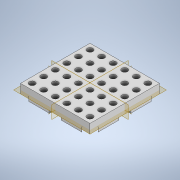
# Autodesk Inventor part: Tile
Saved by Autodesk Inventor 2022.4 (Build 264492010, 492A)
## iProperties
Created: 2025-02-20
Part Number: Tile
Material: Generic
Document SubType Name: Modeling
Designer: jan-m
Density: 1 g/cm^3
Appearance: Default
Author: jan-m
Autodesk Inventor part; units mm, degrees
sketch "Sketch1" plane through (0, 0, 0) normal (0, 1, 0) x (-1, 0, 0)
  line L0 (30, -30) -> (-30, -30)
  line L1 (-30, -30) -> (-30, 30)
  line L2 (-30, 30) -> (30, 30)
  line L3 (30, 30) -> (30, -30)
  line L4 (0, -42) -> (0, 42) projected
  line L5 (-42, 0) -> (42, 0) projected
  point P0 (0, 0)
  point P1 (0, -30)
  point P2 (30, 0)
  dimension "d0" = 60
  dimension "d1" = 60
  constraints: 8 end point, 2 midpoint, 2 parallel, 2 point on line, 1 horizontal, 1 perpendicular
  measures "d0" distance of L0.start L0.end
  measures "d1" distance of L2.end L0.start
extrude "Extrusion1" add sketch "Sketch1" along normal mid plane 10
sketch "Sketch2" plane through (0, -5, 0) normal (0, -1, 0) x (1, 0, 0)
  line L0 (-30, -30) -> (-30, 30) projected
  line L1 (-30, 5) -> (-22, 5)
  line L2 (-22, 5) -> (-22, -5)
  line L3 (-22, -5) -> (-30, -5)
  line L4 (-30, -5) -> (-30, 5)
  arc A0 (-22, -5) -> (-22, 5) centre (-22, 0) ccw
  line L5 (-53.2, 0) -> (53.2, 0) projected
  line L6 (-25, 5) -> (-25, -5)
  line L7 (0, -53.2) -> (0, 53.2) projected
  line L8 (-5, -30) -> (-5, -22)
  arc A1 (5, -22) -> (-5, -22) centre (0, -22) ccw
  line L9 (5, -22) -> (5, -30)
  line L10 (5, -30) -> (-5, -30)
  line L11 (-5, -25) -> (5, -25)
  line L12 (-5, -22) -> (5, -22)
  line L13 (30, -5) -> (22, -5)
  arc A2 (22, 5) -> (22, -5) centre (22, 0) ccw
  line L14 (22, 5) -> (30, 5)
  line L15 (30, 5) -> (30, -5)
  line L16 (25, -5) -> (25, 5)
  line L17 (22, -5) -> (22, 5)
  line L18 (5, 30) -> (5, 22)
  arc A3 (-5, 22) -> (5, 22) centre (0, 22) ccw
  line L19 (-5, 22) -> (-5, 30)
  line L20 (-5, 30) -> (5, 30)
  line L21 (5, 25) -> (-5, 25)
  line L22 (5, 22) -> (-5, 22)
  line L23 (30, -30) -> (-30, -30) projected
  line L24 (30, 30) -> (30, -30) projected
  line L25 (30, -30) -> (24.3431, -24.3431)
  line L26 (30, -30) -> (38, -30) construction
  line L27 (20.8076, -27.8787) -> (22.9289, -30)
  line L28 (27.8787, -20.8076) -> (30, -22.9289)
  line L29 (24.3431, -24.3431) -> (27.8787, -20.8076)
  line L30 (24.3431, -24.3431) -> (20.8076, -27.8787)
  line L31 (22.9289, -30) -> (30, -22.9289)
  line L32 (22.9289, -30) -> (30, -30)
  line L33 (30, -22.9289) -> (30, -30)
  arc A4 (27.8787, -20.8076) -> (20.8076, -27.8787) centre (24.3431, -24.3431) ccw
  line L34 (27.8787, 20.8076) -> (30, 22.9289)
  line L35 (24.3431, 24.3431) -> (27.8787, 20.8076)
  arc A5 (20.8076, 27.8787) -> (27.8787, 20.8076) centre (24.3431, 24.3431) ccw
  line L36 (24.3431, 24.3431) -> (20.8076, 27.8787)
  line L37 (20.8076, 27.8787) -> (22.9289, 30)
  line L38 (22.9289, 30) -> (30, 30)
  line L39 (30, 30) -> (24.3431, 24.3431)
  line L40 (30, 22.9289) -> (22.9289, 30)
  line L41 (30, 22.9289) -> (30, 30)
  line L42 (-20.8076, 27.8787) -> (-22.9289, 30)
  line L43 (-24.3431, 24.3431) -> (-20.8076, 27.8787)
  arc A6 (-27.8787, 20.8076) -> (-20.8076, 27.8787) centre (-24.3431, 24.3431) ccw
  line L44 (-24.3431, 24.3431) -> (-27.8787, 20.8076)
  line L45 (-27.8787, 20.8076) -> (-30, 22.9289)
  line L46 (-30, 22.9289) -> (-30, 30)
  line L47 (-30, 30) -> (-24.3431, 24.3431)
  line L48 (-22.9289, 30) -> (-30, 22.9289)
  line L49 (-22.9289, 30) -> (-30, 30)
  line L50 (-27.8787, -20.8076) -> (-30, -22.9289)
  line L51 (-24.3431, -24.3431) -> (-27.8787, -20.8076)
  arc A7 (-20.8076, -27.8787) -> (-27.8787, -20.8076) centre (-24.3431, -24.3431) ccw
  line L52 (-24.3431, -24.3431) -> (-20.8076, -27.8787)
  line L53 (-20.8076, -27.8787) -> (-22.9289, -30)
  line L54 (-22.9289, -30) -> (-30, -30)
  line L55 (-30, -30) -> (-24.3431, -24.3431)
  line L56 (-30, -22.9289) -> (-22.9289, -30)
  line L57 (-30, -22.9289) -> (-30, -30)
  point P0 (0, 0)
  point P1 (-30, 0)
  point P2 (0, -30)
  point P3 (30, 0)
  point P4 (0, 30)
  point P5 (-30, -5)
  point P6 (20.8076, -20.8076)
  point P7 (20.8076, 20.8076)
  point P8 (-20.8076, 20.8076)
  point P9 (-20.8076, -20.8076)
  dimension "d4" = 10
  dimension "d5" = 8
  dimension "d6" = 3
  dimension "d9" = 360
  dimension "d33" = 135
  dimension "d34" = 5
  dimension "d35" = 5
  dimension "d37" = 8
  dimension "d38" = 3
  dimension "d39" = 7.0711
  dimension "d45" = 5
  dimension "d48" = 360
  constraints: 110 end point, 32 point on line, 20 point on circle, 8 centre point, 4 perpendicular, 2 horizontal, 2 parallel, 2 tangent, 1 equal length, 1 midpoint, 142 other
  measures "d4" distance between parallel lines of L3 L1
  measures "d5" distance of L1.start L1.end
  measures "d6" distance between parallel lines of L2 L6
  measures "d33" angle of L26 L25
  measures "d34" distance between parallel lines of L25 L27
  measures "d35" distance between parallel lines of L25 L28
  measures "d37" distance of L23.start L25.end
  measures "d38" distance between parallel lines of L31 L30
  measures "d39" distance of A4.start point (20.808, -20.808)
  measures "d45" radius of A4
extrude "Extrusion2" cut sketch "Sketch2" against normal blind 2 contours L0 L47 L48 | L40 L39 L24 | L55 L56 L23 | L0 L56 L55 | L0 L5 L6 L3 | L8 L11 L7 L10 | L0 L1 L6 L5 | L7 L11 L9 L10 | L31 L25 L23 | L49 L48 L47 | L25 L31 L24 | L13 L16 L5 L15 | L16 L14 L15 L5 | L21 L19 L20 L7 | L7 L20 L18 L21 | L39 L40 L38
extrude "Extrusion3" cut sketch "Sketch2" against normal blind 4 contours L48 L47 L44 L45 | A3 L22 L7 | L7 L22 A3 | L34 L35 L39 L40 | L50 L51 L55 L56 | L56 L55 L52 L53 | A7 L52 L51 | L6 L5 L2 L3 | L8 L12 L7 L11 | L6 L1 L2 L5 | L2 L5 A0 | A1 L7 L12 | L7 L12 L9 L11 | L2 A0 L5 | A1 L12 L7 | L27 L30 L25 L31 | L44 L43 A6 | L48 L42 L43 L47 | A4 L29 L30 | L25 L29 L28 L31 | A2 L17 L5 | L5 L17 A2 | L17 L14 L16 L5 | L5 L16 L13 L17 | L22 L19 L21 L7 | L7 L21 L18 L22 | A5 L36 L35 | L39 L36 L37 L40
sketch "Sketch3" plane through (0, 5, 0) normal (0, 1, 0) x (1, 0, 0)
  circle A0 centre (-25, 25) radius 2.5
  line L0 (30, 30) -> (-30, 30) projected
  line L1 (-30, 30) -> (-30, -30) projected
  line L2 (-42, 0) -> (42, 0) projected
  line L3 (0, 42) -> (0, -42) projected
  circle A1 centre (-25, 15) radius 2.5
  circle A2 centre (-25, 5) radius 2.5
  circle A3 centre (-25, -5) radius 2.5
  circle A4 centre (-25, -15) radius 2.5
  circle A5 centre (-15, 25) radius 2.5
  circle A6 centre (-15, 15) radius 2.5
  circle A7 centre (-15, 5) radius 2.5
  circle A8 centre (-15, -5) radius 2.5
  circle A9 centre (-15, -15) radius 2.5
  circle A10 centre (-5, 25) radius 2.5
  circle A11 centre (-5, 15) radius 2.5
  circle A12 centre (-5, 5) radius 2.5
  circle A13 centre (-5, -5) radius 2.5
  circle A14 centre (-5, -15) radius 2.5
  circle A15 centre (5, 25) radius 2.5
  circle A16 centre (5, 15) radius 2.5
  circle A17 centre (5, 5) radius 2.5
  circle A18 centre (5, -5) radius 2.5
  circle A19 centre (5, -15) radius 2.5
  circle A20 centre (15, 25) radius 2.5
  circle A21 centre (15, 15) radius 2.5
  circle A22 centre (15, 5) radius 2.5
  circle A23 centre (15, -5) radius 2.5
  circle A24 centre (15, -15) radius 2.5
  circle A25 centre (-25, -25) radius 2.5
  circle A26 centre (-15, -25) radius 2.5
  circle A27 centre (-5, -25) radius 2.5
  circle A28 centre (5, -25) radius 2.5
  circle A29 centre (15, -25) radius 2.5
  circle A30 centre (25, 25) radius 2.5
  circle A31 centre (25, 15) radius 2.5
  circle A32 centre (25, 5) radius 2.5
  circle A33 centre (25, -5) radius 2.5
  circle A34 centre (25, -15) radius 2.5
  circle A35 centre (25, -25) radius 2.5
  point P0 (0, 0)
  dimension "d15" = 5
  dimension "d16" = 5
  dimension "d17" = 5
  dimension "d20" = 10
  dimension "d23" = 10
  constraints: 36 centre point, 1 horizontal, 1 vertical, 70 other
  measures "d15" diameter of A0
  measures "d16" distance from line of L0 A0.centre
  measures "d17" distance from line of L1 A0.centre
  measures "d20" distance of A0.centre A1.centre
  measures "d23" distance of A0.centre A5.centre
extrude "Extrusion4" cut sketch "Sketch3" against normal blind 5 contours A0 | A1 | A2 | A3 | A4 | A5 | A6 | A7 | A8 | A9 | A10 | A11 | A12 | A13 | A14 | A15 | A16 | A17 | A18 | A19 | A20 | A21 | A22 | A23 | A24 | A25 | A26 | A27 | A28 | A29 | A30 | A31 | A32 | A33 | A34 | A35
body "Solid1"
